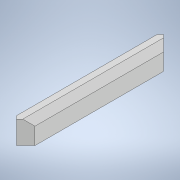
# Autodesk Inventor part: outside-join-2
Saved by Autodesk Inventor 2021 (Build 250183000, 183)
## iProperties
Created: 2020-12-08
Part Number: outside-join-2
Material: Generic
Document SubType Name: Modeling
Designer: Luke Kamols
Density: 1 g/cm^3
Appearance: Default
Author: Luke Kamols
Autodesk Inventor part; units mm, degrees
ref_plane "YZ Plane" through (0, 0, 0) normal (1, 0, 0) x (0, 1, 0)
ref_plane "XZ Plane" through (0, 0, 0) normal (0, 1, 0) x (-1, 0, 0)
ref_plane "XY Plane" through (0, 0, 0) normal (0, 0, 1) x (1, 0, 0)
sketch "Sketch1" plane through (0, 0, 0) normal (0, 0, 1) x (1, 0, 0)
  line L0 (6, 0) -> (6, 11)
  line L1 (0, 15) -> (2, 15)
  line L2 (2, 15) -> (6, 11)
  line L3 (0, 10) -> (3, 7)
  line L4 (-6, 0) -> (-6, 11)
  line L5 (0, 15) -> (-2, 15)
  line L6 (-2, 15) -> (-6, 11)
  line L7 (0, 10) -> (-3, 7)
  line L8 (-4.5, 0) -> (-3, 7)
  line L9 (3, 7) -> (4.5, 0)
  line L10 (-6, 0) -> (-4.5, 0)
  line L11 (4.5, 0) -> (6, 0)
  point P0 (0, 0)
  dimension "d2" = 11
  dimension "d4" = 2
  dimension "d5" = 10
  constraints: 24 end point, 1 collinear, 1 horizontal
  measures "d2" distance of L0.start L0.end
  measures "d4" distance of L1.start L1.end
  measures "d5" distance of point (0, 0) L3.start
extrude "Extrusion1" add sketch "Sketch1" along normal blind 66
sketch "Sketch2" plane through (0, 0, 66) normal (0, 0, 1) x (1, 0, 0)
  line L0 (2, 15) -> (-2, 15) projected
  line L1 (0, 15) -> (2, 15)
  line L2 (6, 11) -> (2, 15) projected
  line L3 (4.5, 0) -> (6, 0) projected
  line L4 (0, 0) -> (6, 0)
  line L5 (6, 0) -> (6, 11) projected
  line L6 (6, 0) -> (6, 11)
  line L7 (6, 11) -> (2, 15)
  line L8 (0, 15) -> (-2, 15)
  line L9 (-2, 15) -> (0, 0)
  constraints: 12 end point, 2 collinear, 1 horizontal, 1 midpoint, 1 perpendicular, 1 point on line
extrude "Extrusion2" add sketch "Sketch2" along normal blind 15
sketch "Sketch5" plane through (0, 0, 0) normal (0, 0, -1) x (-1, 0, 0)
  line L0 (0, 0) -> (-6, 0) projected
  line L1 (-6, 0) -> (-6, 11) projected
  line L2 (-6, 11) -> (-2, 15) projected
  line L3 (-2, 15) -> (2, 15) projected
  line L4 (2, 15) -> (0, 0) projected
extrude "Extrusion4" add sketch "Sketch5" along normal blind 15
sketch "Sketch6" plane through (0, 0, 66) normal (0, -1, 0) x (1, 0, 0)
  line L0 (0, -66) -> (0, -81) projected
  line L1 (6, -81) -> (6, 15) projected
  line L2 (0, -81) -> (6, -81)
  line L3 (6, -81) -> (6, -75)
  line L4 (6, -75) -> (0, -81)
  line L5 (-2, -81) -> (2, -81) projected
  line L6 (0, -81) -> (-2, -81)
  line L7 (-2, -81) -> (-2, -79)
  line L8 (-2, -66) -> (-2, -81) projected
  line L9 (-2, -79) -> (0, -81)
  line L10 (2, 15) -> (-2, 15) projected
  line L11 (6, 15) -> (2, 15) projected
  line L12 (0, 15) -> (6, 15)
  line L13 (6, 15) -> (6, 9)
  line L14 (0, 0) -> (0, 15) projected
  line L15 (6, 9) -> (0, 15)
  line L16 (0, 15) -> (-2, 15)
  line L17 (-2, 0) -> (-2, 15) projected
  line L18 (-2, 15) -> (-2, 13)
  line L19 (-2, 13) -> (0, 15)
  dimension "d16" = 6
  dimension "d17" = 2
  dimension "d18" = 6
  constraints: 24 end point, 4 horizontal, 4 point on line, 1 midpoint
  measures "d16" distance of L1.start L3.end
  measures "d17" distance of L5.start L7.end
  measures "d18" distance of L1.end L13.end
extrude "Extrusion5" cut sketch "Sketch6" against normal blind 37.3875
body "Solid1"
